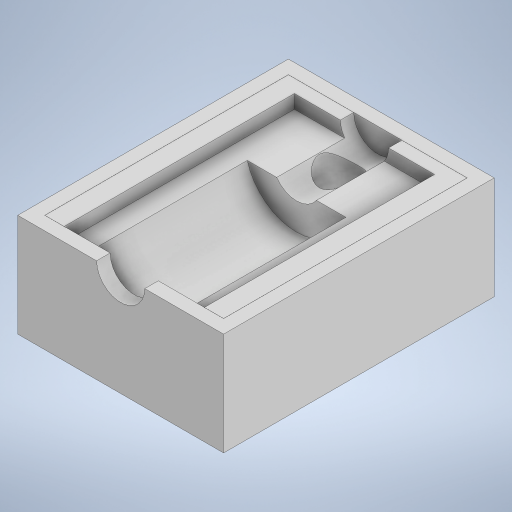
# Autodesk Inventor part: gen housing
Saved by Autodesk Inventor 2024 (Build 280153000, 153)
## iProperties
Created: 2024-05-21
Part Number: gen housing
Material: Generic
Document SubType Name: Sheet Metal
Designer: albah
Density: 1 g/cm^3
Sheet Metal Rule: Default_mm
Appearance: Default
Author: albah
Autodesk Inventor part; units mm, degrees
ref_plane "YZ Plane" through (0, 0, 0) normal (1, 0, 0) x (0, 1, 0)
ref_plane "XZ Plane" through (0, 0, 0) normal (0, 1, 0) x (-1, 0, 0)
ref_plane "XY Plane" through (0, 0, 0) normal (0, 0, 1) x (1, 0, 0)
sketch "Sketch1" plane through (0, 0, 0) normal (0, 0, 1) x (1, 0, 0)
  line L0 (11.305, 0) -> (48.3, 0)
  line L1 (48.3, 0) -> (48.3, -48.3)
  line L2 (48.3, -48.3) -> (0, -48.3)
  arc A0 (0, -11.305) -> (11.305, 0) centre (0, 0) ccw
  line L3 (-11.305, 0) -> (-48.3, 0)
  line L4 (-48.3, 0) -> (-48.3, -48.3)
  line L5 (-48.3, -48.3) -> (0, -48.3)
  arc A1 (-11.305, 0) -> (0, -11.305) centre (0, 0) ccw
  dimension "d0" = 48.3
  dimension "d1" = 48.3
  constraints: 12 end point, 4 point on circle, 2 centre point, 2 coincident, 1 horizontal, 1 parallel, 1 perpendicular
  measures "d0" distance of point (0, 0) L0.end
  measures "d1" distance of L0.end L1.end
extrude "Extrusion1" add sketch "Sketch1" against normal blind 127
sketch "Sketch4" plane through (0, 0, 0) normal (0, 0, 1) x (1, 0, 0)
  line L0 (11.305, 0) -> (48.3, 0) projected
  line L1 (11.305, 0) -> (17.655, 0)
  line L2 (17.655, -9.652) -> (5.8857, -9.652)
  arc A0 (-11.305, 0) -> (11.305, 0) centre (0, 0) ccw projected
  line L3 (17.655, 0) -> (24.005, 0)
  line L4 (24.005, 0) -> (24.005, -9.652)
  line L5 (24.005, -9.652) -> (17.655, -9.652)
  line L6 (-17.655, -9.652) -> (-5.8857, -9.652)
  line L7 (-24.005, 0) -> (-24.005, -9.652)
  line L8 (-24.005, -9.652) -> (-17.655, -9.652)
  constraints: 16 end point, 2 point on line, 1 perpendicular, 1 point on circle, 1 vertical
shell "Shell1" thickness 6.35 removed faces 4 at (-23.6367, 0, -42.3333) at (35.9683, 0, -42.3333) at (-10.8028, -3.3322, -84.6667) at (3.3322, -10.8028, -84.6667)
sketch "Sketch5" plane through (-41.95, -41.95, -6.35) normal (0, 1, 0) x (1, 0, 0)
  line L0 (30.645, 114.3) -> (30.645, 120.65) projected
  line L1 (53.255, 0) -> (30.645, 0) projected
  line L2 (30.645, 114.3) -> (30.645, 0)
  line L3 (30.645, 0) -> (53.255, 0)
  line L4 (53.255, 0) -> (53.255, 114.3)
  line L5 (53.255, 114.3) -> (30.645, 114.3)
  line L6 (30.645, 0) -> (17.945, 0)
  line L7 (17.945, 0) -> (17.945, 114.3)
  line L8 (17.945, 114.3) -> (30.645, 114.3)
  line L9 (30.645, 0) -> (17.945, 0)
  line L10 (17.945, 88.8975) -> (30.645, 88.8975)
  line L11 (30.645, 114.3) -> (53.255, 114.3)
  line L12 (53.255, 114.3) -> (53.255, 120.65) projected
  line L13 (30.645, 120.65) -> (53.255, 120.65) projected
  line L14 (53.255, 120.65) -> (30.645, 120.65)
  line L15 (30.645, 120.65) -> (30.645, 114.3)
  circle A0 centre (41.95, 95.9615) radius 9.0868
  line L16 (0, 114.3) -> (30.645, 114.3) projected
  line L17 (0, 0) -> (83.9, 0) projected
  line L18 (0, 114.3) -> (83.9, 114.3)
  line L19 (83.9, 114.3) -> (83.9, 0)
  line L20 (83.9, 0) -> (0, 0)
  line L21 (0, 0) -> (0, 114.3)
  line L22 (53.255, 114.3) -> (53.255, 0)
  line L23 (65.955, 0) -> (65.955, 114.3)
  line L24 (65.955, 114.3) -> (53.255, 114.3)
  line L25 (65.955, 88.8975) -> (53.255, 88.8975)
  point P0 (41.95, -6.35)
  dimension "d21" = 12.7
  constraints: 40 end point, 9 perpendicular, 6 point on line, 3 parallel, 1 centre point, 1 collinear, 1 horizontal, 1 vertical
  measures "d21" distance of L1.end L6.end
extrude "Extrusion2" add sketch "Sketch5" along normal blind 41.91 contours L5 L4 L1 L2
hole "Hole1" at (0, 0, 0) direction (0, 0, -1) diameter 22.606 end through all
sketch "Sketch8" plane through (-41.95, -41.95, -6.35) normal (0, 1, 0) x (1, 0, 0)
  line L0 (30.645, -6.35) -> (30.645, 0) projected
  line L1 (30.645, 0) -> (30.645, 89.0193)
  line L2 (30.645, 114.3) -> (30.645, 0) projected
  line L3 (0, 0) -> (0, 114.3) projected
  line L4 (0, 89.0193) -> (0, 114.3)
  line L5 (0, 114.3) -> (30.645, 114.3)
  line L6 (30.645, 114.3) -> (30.645, 89.0193)
  line L7 (0, 89.0193) -> (30.645, 89.0193)
  line L8 (-6.35, -6.35) -> (-6.35, 120.65) projected
  line L9 (30.645, 89.0193) -> (30.645, 114.3)
  line L10 (53.2529, 114.3) -> (53.2529, 0) projected
  line L11 (53.2529, 89.0193) -> (83.9, 89.0193)
  line L12 (83.9, 114.3) -> (83.9, 0) projected
  line L13 (83.9, 114.3) -> (53.2529, 114.3)
  line L14 (53.2529, 114.3) -> (53.2529, 89.0193)
  point P0 (41.95, -6.35)
  constraints: 18 end point, 5 perpendicular, 5 point on line, 2 horizontal, 1 collinear
extrude "Extrusion3" add sketch "Sketch8" along normal blind 41.91
sketch "Sketch13" plane through (11.305, -41.95, -6.35) normal (0, 1, 0) x (1, 0, 0)
  line L0 (-53.255, 0) -> (-53.255, 89.0193) projected
  line L1 (-53.255, 0) -> (-22.61, 0) projected
  line L2 (-53.255, 89.0193) -> (-22.61, 89.0193)
  line L3 (-22.61, 89.0193) -> (-22.61, 0)
  line L4 (-22.61, 0) -> (-53.255, 0)
  line L5 (-53.255, 0) -> (-53.255, 89.0193)
  line L6 (0, 89.0193) -> (0, 0) projected
  line L7 (30.645, 0) -> (30.645, 89.0193) projected
  line L8 (0, 89.0193) -> (30.645, 89.0193)
  line L9 (30.645, 89.0193) -> (30.645, 0)
  line L10 (30.645, 0) -> (0, 0)
  line L11 (0, 0) -> (0, 89.0193)
  line L12 (0, 89.0193) -> (12.7, 89.0193)
  line L13 (30.645, 89.0193) -> (0, 89.0193) projected
  line L14 (0, 0) -> (12.7, 0)
  line L15 (12.7, 0) -> (12.7, 89.0193)
  line L16 (12.7, 89.0193) -> (0, 89.0193)
  line L17 (0, 89.0193) -> (0, 0)
  line L18 (0, 89.0193) -> (-12.7, 89.0193)
  line L19 (0, 0) -> (-12.7, 0)
  line L20 (-12.7, 0) -> (-12.7, 89.0193)
  line L21 (-22.61, 120.65) -> (0, 120.65) projected
  line L22 (-22.6079, 114.3) -> (-0.0021, 114.3) projected
  line L23 (-22.61, 89.0193) -> (-22.61, 0)
  line L24 (-22.61, 0) -> (-35.31, 0)
  line L25 (-35.31, 0) -> (-35.31, 89.0193)
  line L26 (-35.31, 89.0193) -> (-22.61, 89.0193)
  constraints: 40 end point, 6 parallel, 3 horizontal, 3 perpendicular, 2 symmetric about line, 1 point on line
extrude "Extrusion6" add sketch "Sketch13" along normal blind 41.91 contours L0 L2 L25 L1 | L8 L7 L10 L15
sketch "Sketch18" plane through (-11.305, -41.95, -6.35) normal (0, 1, 0) x (1, 0, 0)
  line L0 (0.0021, 0) -> (0.0021, 114.3) projected
  line L1 (-12.7, 0) -> (-12.7, 89.0193) projected
  line L2 (0.0021, 0) -> (-12.7, 0)
  line L3 (-12.7, 0) -> (-12.7, 89.0193)
  line L4 (-12.7, 89.0193) -> (0.0021, 89.0193)
  line L5 (0.0021, 89.0193) -> (0.0021, 0)
  line L6 (35.31, 89.0193) -> (35.31, 0) projected
  line L7 (22.608, 0) -> (35.31, 0)
  line L8 (35.31, 0) -> (35.31, 89.0193)
  line L9 (35.31, 89.0193) -> (22.608, 89.0193)
  line L10 (22.608, 89.0193) -> (22.608, 0)
  point P0 (11.305, -6.35)
  point P1 (35.31, 0)
  constraints: 16 end point, 4 parallel, 2 horizontal, 2 perpendicular, 1 point on line
extrude "Extrusion7" add sketch "Sketch18" along normal blind 35.56
sketch "Sketch19" plane through (-11.305, -0.04, -95.3693) normal (-1, 0, 0) x (0, 0, 1)
  line L0 (0, 0) -> (89.0193, 0) projected
  line L1 (89.0193, 0) -> (89.0193, -6.35) projected
  line L2 (0, 0) -> (89.0193, 0)
  line L3 (89.0193, 0) -> (89.0193, -6.35)
  line L4 (89.0193, -6.35) -> (0, -6.35)
  line L5 (0, -6.35) -> (0, 0)
  point P0 (95.3693, 0.04)
  constraints: 8 end point, 2 parallel, 1 horizontal, 1 perpendicular
extrude "Extrusion8" cut sketch "Sketch19" against normal blind 25.4
sketch "Sketch20" plane through (0, 0, -127) normal (0, 0, -1) x (-1, 0, 0)
  arc A0 (-11.305, 0) -> (11.305, 0) centre (0, 0) ccw projected
  arc A1 (-11.305, 0) -> (0, -11.305) centre (0, 0) ccw
  line L0 (11.305, 0) -> (-11.305, 0)
  constraints: 3 point on circle, 2 end point, 1 centre point, 1 coincident, 1 horizontal
extrude "Extrusion9" add sketch "Sketch20" against normal blind 6.35
sketch "Sketch23" plane through (41.95, 0, -6.35) normal (0, 0, -1) x (-1, 0, 0)
  circle A0 centre (41.95, 0) radius 24.005
  point P0 (65.955, -0.04)
  constraints: 1 coincident, 3 other
extrude "Extrusion10" cut sketch "Sketch23" along normal blind 76.2
move faces "Move1" translate (8.89, 0, 0) faces at (24.005, -4.2733, -65.6962)
move faces "Move2" translate (-8.89, 0, 0) faces at (-24.005, -4.2733, -36.0231)
delete faces "Delete1" heal yes whole lump no faces at (-1.0741, -41.95, -99.4794)
move faces "Move3" translate (0, 0, -19.05) faces at (-25.6206, -2.9016, -95.3693)
move faces "Move4" translate (0, 0, -19.05) faces at (25.6206, -2.9016, -95.3693)
equation "\"d29\" = Thickness"
equation "\"BendRadius\" = Thickness"
equation "\"BendReliefWidth\" = Thickness"
equation "\"BendReliefDepth\" = 0.5 * Thickness"
equation "\"CornerReliefSize\" = 4 * Thickness"
equation "\"MinimumRemnant\" = 2 * Thickness"
equation "\"TransitionRadius\" = BendRadius"
equation "\"JacobiRadiusSize\" = BendRadius"
equation "\"GapSize\" = Thickness"
equation "\"Thickness\" = 0.5"
body "Solid1"
